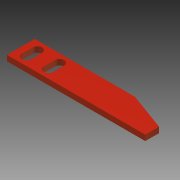
# Autodesk Inventor part: 13_0204_068
Saved by Autodesk Inventor 2012 SP1 (Build 160190100, 190)
## iProperties
Created: 2013-04-30
Part Number: 13_0204_068
Material: Default
Document SubType Name: Modeling
Designer: vogel
Density: 1 g/cm^3
Author: vogel
Autodesk Inventor part; units mm, degrees
ref_plane "YZ Plane" through (0, 0, 0) normal (1, 0, 0) x (0, 1, 0)
ref_plane "XZ Plane" through (0, 0, 0) normal (0, 1, 0) x (-1, 0, 0)
ref_plane "XY Plane" through (0, 0, 0) normal (0, 0, 1) x (1, 0, 0)
sketch "Skizze1" plane through (0, 0, 0) normal (0, 0, 1) x (1, 0, 0)
  line L0 (0, 0) -> (50, 0)
  line L1 (50, 0) -> (50, 5)
  line L2 (36.2626, 10) -> (0, 10)
  line L3 (0, 10) -> (0, 0)
  line L4 (36.2626, 10) -> (50, 5)
  dimension "d0" = 10
  dimension "d1" = 50
  dimension "d2" = 5
  dimension "d5" = 20
  constraints: 10 end point, 2 parallel, 1 horizontal, 1 perpendicular
  measures "d0" distance of L2.end L0.start
  measures "d1" distance of L0.start L0.end
  measures "d2" distance of L0.end L1.end
  measures "d5" angle of L4 L2
extrude "Extrusion1" add sketch "Skizze1" along normal blind 2
sketch "Skizze2" plane through (0, 0, 2) normal (0, 0, 1) x (1, 0, 0)
  line L0 (0, 0) -> (0, 10) projected
  line L1 (0, 10) -> (36.2626, 10) projected
  line L2 (0, 5) -> (28.2614, 5)
  point P0 (4, 5)
  point P1 (12, 5)
  dimension "d8" = 4
  dimension "d9" = 8
  constraints: 2 end point, 2 point on line, 1 midpoint, 1 parallel
  measures "d8" distance from line of L0 point (4, 5)
  measures "d9" distance of point (12, 5) point (4, 5)
hole "Bohrung1" at (4, 5, 2) at (12, 5, 2) direction (0, 0, -1) diameter 3.4 end through all
sketch "Skizze4" plane through (0, 0, 2) normal (0, 0, 1) x (1, 0, 0)
  circle A0 centre (4, 5) radius 1.7 projected
  line L0 (50, 0) -> (0, 0) projected
  line L1 (0, 10) -> (36.2626, 10) projected
  line L2 (5.7, 7) -> (5.7, 3)
  line L3 (2.3, 3) -> (2.3, 7)
  arc A1 (5.7, 7) -> (2.3, 7) centre (4, 7) ccw
  arc A2 (2.3, 3) -> (5.7, 3) centre (4, 3) ccw
  dimension "d17" = 3
  dimension "d18" = 3
  dimension "d19" = 4
  constraints: 6 tangent, 4 end point, 4 point on circle, 2 centre point, 1 parallel, 1 vertical
  measures "d17" distance from line of A2.centre L0
  measures "d18" distance from line of L1 A1.centre
  measures "d19" distance of A1.centre A2.centre
extrude "Extrusion2" cut sketch "Skizze4" against normal through all contours L2 A2 L3 A0 | A0 L3 A1 L2
pattern_linear "Rechteckige Anordnung1" count 2 spacing 8 along (1, 0, 0) of "Extrusion2"
